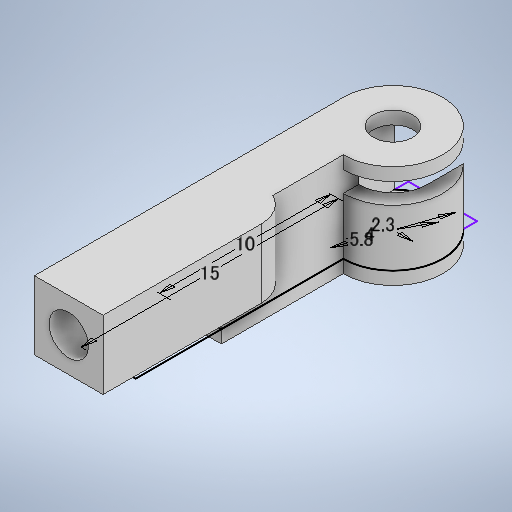
# Autodesk Inventor part: srod1.3
Saved by Autodesk Inventor 2025 (Build 290162000, 162)
## iProperties
Created: 2024-07-28
Part Number: srod1.3
Material: 一般
Document SubType Name: Modeling
Designer: Saigusa
Density: 1 g/cm^3
Appearance: 既定
Author: Saigusa
Autodesk Inventor part; units mm, degrees
ref_plane "YZ Plane" through (0, 0, 0) normal (1, 0, 0) x (0, 1, 0)
ref_plane "XZ Plane" through (0, 0, 0) normal (0, 1, 0) x (-1, 0, 0)
ref_plane "XY Plane" through (0, 0, 0) normal (0, 0, 1) x (1, 0, 0)
sketch "スケッチ1" plane through (0, 0, 0) normal (0, 1, 0) x (-1, 0, 0)
  circle A0 centre (0, 0) radius 1.15
  circle A1 centre (0, 0) radius 2
  circle A2 centre (0, 0) radius 2.9
  line L0 (-2, 0) -> (2, 0)
  line L1 (2, 0) -> (2, -2.9)
  line L2 (2, -2.9) -> (-2, -2.9)
  line L3 (-2, -2.9) -> (-2, 0)
  line L4 (0, 0) -> (0, 2.9)
  line L5 (0, 0) -> (2.9, 0)
  line L6 (2.9, 0) -> (2.9, 15)
  line L7 (2.9, 15) -> (0, 15)
  line L8 (0, 15) -> (0, 0)
  line L9 (0, 0) -> (2.9, 0)
  line L10 (2.9, 0) -> (2.9, 10)
  line L11 (2.9, 10) -> (0, 10)
  line L12 (0, 10) -> (0, 0)
  point P0 (0, 2)
  point P1 (-2, -2.1)
  point P2 (2, -2.1)
  dimension "d1" = 4
  dimension "d2" = 5.8
  dimension "d0" = 2.3
  dimension "d3" = 15
  dimension "d4" = 10
  constraints: 26 end point, 6 parallel, 3 coincident, 3 horizontal, 3 perpendicular, 1 centre point, 1 point on line, 1 vertical, 6 other
  measures "d0" diameter of A0
  measures "d3" distance of L6.end L5.end
  measures "d4" distance of L10.end L9.end
extrude "押し出し1" add sketch "スケッチ1" along normal blind 3.3 contours A1 L3 A2 L4
extrude "押し出し2" add sketch "スケッチ1" along normal blind 4.5 contours L5 A2 L1 | A1 L4 A2 L5 | A2 L8 L11 L6
extrude "押し出し3" add sketch "スケッチ1" against normal blind 0.75 contours L0 A1 A0 | A0 L4 A1 L0 | A0 L0 A1 L4 | L1 A2 L3 A1 | L5 A2 L1 | A1 L4 A2 L5 | A1 L3 A2 L4 | A2 L8 L11 L6
sketch "スケッチ2" plane through (0, 4.5, 0) normal (0, 1, 0) x (1, 0, 0)
  circle A0 centre (0, 0) radius 1.15
  line L0 (-2, 0) -> (-2, 2.1) projected
  circle A1 centre (0, 0) radius 2
  arc A2 (-2, 2.1) -> (-2.9, 0) centre (0, 0) ccw projected
  circle A3 centre (0, 0) radius 2.9
  line L1 (-2, 0) -> (2, 0)
  line L2 (2, 0) -> (2, 2.9)
  line L3 (2, 2.9) -> (-2, 2.9)
  line L4 (-2, 2.9) -> (-2, 0)
  line L5 (-2.9, 0) -> (-2.9, -10) projected
  line L6 (-2.9, -10) -> (0, -10) projected
  line L7 (-2.9, 0) -> (0, 0)
  line L8 (0, 0) -> (0, -10)
  line L9 (0, -10) -> (-2.9, -10)
  line L10 (-2.9, -10) -> (-2.9, 0)
  point P0 (0, -2.9)
  constraints: 16 end point, 4 parallel, 3 coincident, 2 horizontal, 2 perpendicular, 1 centre point, 1 horizontal alignment, 5 other
extrude "押し出し4" add sketch "スケッチ2" along normal blind 0.75 contours L1 A1 L8 A0 | A0 L1 A1 | A0 L8 A1 L1 | L2 A3 L8 A1 | A1 L0 A3 L2 | L7 A2 L0 | A1 L8 A3 L7 | A3 L8 L6 L5
sketch "スケッチ3" plane through (-2.9, -0.75, 10) normal (0, 0, 1) x (1, 0, 0)
  line L0 (4.05, 0) -> (1.75, 0) projected
  line L1 (0, 0) -> (0, 6) projected
  line L2 (2.9, 0) -> (0, 0)
  line L3 (0, 0) -> (0, 0.75)
  line L4 (0, 0.75) -> (2.9, 0.75)
  line L5 (2.9, 0.75) -> (2.9, 0)
  line L6 (2.9, 0.75) -> (1.4, 0.75)
  line L7 (1.4, 0.75) -> (1.4, 1.15)
  line L8 (1.4, 1.15) -> (2.9, 1.15)
  line L9 (2.9, 1.15) -> (2.9, 0.75)
  line L10 (1.4, 0.75) -> (1.4, 1.25)
  dimension "d13" = 1.5
  dimension "d14" = 0.4
  dimension "d15" = 0.5
  constraints: 18 end point, 4 parallel, 2 horizontal, 2 perpendicular, 1 midpoint, 1 point on line, 1 vertical
  measures "d13" distance of L7.end L8.end
  measures "d14" distance of L6.end L7.end
  measures "d15" distance of L6.end L10.end
hole "穴1" at (-1.5, 0.5, 10) direction (0, 0, -1) diameter 1 end through all
sketch "スケッチ4" plane through (-2.9, -0.75, 10) normal (0, 0, 1) x (1, 0, 0)
  line L0 (0, 0) -> (0, 6) projected
  line L1 (0, 6) -> (4, 6)
  line L2 (4, 6) -> (4, 2)
  line L3 (4, 2) -> (0, 2)
  line L4 (0, 2) -> (0, 6)
  point P0 (2.9, 0.75)
  dimension "d23" = 4
  dimension "d24" = 4
  constraints: 8 end point, 2 parallel, 1 horizontal, 1 perpendicular
  measures "d23" distance of L2.end L3.end
  measures "d24" distance of L1.end L2.end
extrude "押し出し5" add sketch "スケッチ4" along normal blind 8 and the other way blind 3
sketch "スケッチ5" plane through (-2.9, -0.75, 18) normal (0, 0, 1) x (1, 0, 0)
  line L0 (5.8, 6) -> (0, 6) projected
  line L1 (0, 6) -> (2, 6)
  line L2 (2, 6) -> (2, 4)
  line L3 (2, 4) -> (0, 4)
  line L4 (0, 4) -> (0, 6)
  point P0 (2.9, 0.75)
  point P1 (2.9, 6)
  dimension "d29" = 2
  dimension "d30" = 2
  constraints: 8 end point, 2 parallel, 1 horizontal, 1 perpendicular
  measures "d29" distance of L2.end L3.end
  measures "d30" distance of L1.end L2.end
hole "穴2" at (-0.9, 3.25, 18) direction (0, 0, -1) diameter 2.3 depth 10
fillet "フィレット1" radius 2 1 edges at (1.1, 3.25, 7)
